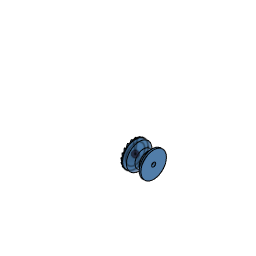
winch (Autodesk Fusion 360 design; units mm, degrees)
Autodesk Fusion 360 part; units mm, degrees
ref_plane "WorkPlane1" through (57.6974, -22.6085, 21.97) normal (-1, 0, 0) x (0, -1, 0)
sketch "Sketch1" plane through (57.6974, -45.4789, 40.4785) normal (-1, 0, 0) x (0, 1, 0)
  circle A0 centre (0, 0) radius 15
  line L0 (0, 0) -> (-2.3758, -15)
  line L1 (-2.3758, -15) -> (2.3758, -15)
  line L2 (2.3758, -15) -> (0, 0)
  circle A1 centre (0, 0) radius 11.1
  dimension "d113" = 30
  dimension "d114" = 18
  constraint coincident A0.centre L0.start
  constraint horizontal L1
  constraint tangent A0 L1
  constraint equal L0 L2
  measures "d113" diameter of A0
  measures "d114" angle of L0 L2
sketch "Sketch3" plane through (57.6974, -45.4789, 40.4785) normal (-1, 0, 0) x (0, 1, 0)
extrude "Extrude1" add sketch "Sketch1" against normal blind 7 contours A0 L0 L2 A1 | A0 L0 L2 A1 makes body 1
ref_plane "WorkPlane2" through (61.033, -45.4789, 55.4785) normal (0, 0, 1) x (0, 1, 0)
extrude "Extrude2" add sketch "Sketch1" along normal blind 2.1974 separate body contours A0 L0 L2 A1 picked at (1.2951, -12.322) makes body 2
sketch "Sketch2" plane through (36.883, -45.4789, 55.4785) normal (0, 0, 1) x (1, 0, 0)
  line L0 (20.8144, 2.3465) -> (18.617, 2.3465) construction
  line L1 (18.617, 2.3465) -> (18.617, -2.3465) construction
  line L2 (18.617, -2.3465) -> (20.8144, -2.3465) construction
  line L3 (18.617, 2.3465) -> (20.8144, -2.3465)
  line L4 (20.8144, -2.3465) -> (18.617, -2.3465)
  line L5 (18.617, -2.3465) -> (18.617, 2.3465)
  line L6 (20.8144, 2.3465) -> (20.8144, -2.3465)
  constraint coincident L0.end L1.start
  constraint coincident L2.end L3.end
  constraint coincident L1.end L2.start
extrude "Extrude3" cut sketch "Sketch2" against normal blind 10 bodies 2
pattern_circular "C-Pattern1" count 20 over 360 about axis through (57.6974, -45.4789, 40.4785) along (1, 0, 0) of bodies 2 makes body 3 at (56.5987, -49.3076, 52.2619) makes body 4 at (56.5987, -52.7615, 50.5021) makes body 5 at (56.5987, -55.5025, 47.761) makes body 6 at (56.5987, -57.2624, 44.3071) makes body 7 at (56.5987, -57.8688, 40.4785) makes body 8 at (56.5987, -57.2624, 36.6498) makes body 9 at (56.5987, -55.5025, 33.1959) makes body 10 at (56.5987, -52.7615, 30.4548) makes body 11 at (56.5987, -49.3076, 28.695) makes body 12 at (56.5987, -45.4789, 28.0886) makes body 13 at (56.5987, -41.6502, 28.695) makes body 14 at (56.5987, -38.1963, 30.4548) makes body 15 at (56.5987, -35.4553, 33.1959) makes body 16 at (56.5987, -33.6954, 36.6498) makes body 17 at (56.5987, -33.089, 40.4785) makes body 18 at (56.5987, -33.6954, 44.3071) makes body 19 at (56.5987, -35.4553, 47.761) makes body 20 at (56.5987, -38.1963, 50.5021) makes body 21 at (56.5987, -41.6502, 52.2619)
combine "Combine1" operation add target body 1 tool bodies 11 7 8 6 5 9 10 2 12 3 4 19 14 17 21 13 15 16 20 18
sketch "Sketch3 (1)" plane through (64.6974, 0, 0) normal (1, 0, 0) x (0, 1, 0)
  circle A0 centre (-45.4789, 40.4785) radius 11.1
  circle A1 centre (-45.4789, 40.4785) radius 15
  circle A2 centre (-45.4789, 40.4785) radius 4.1
  dimension "d144" = 8.2
  constraint concentric A0 A2
  measures "d144" diameter of A2
extrude "Extrude4" add sketch "Sketch3 (1)" along normal blind 2.1974 contours A0 | A1 bodies 1
sketch "Sketch4" plane through (66.8948, 0, 0) normal (1, 0, 0) x (0, 1, 0)
  circle A0 centre (-45.4789, 40.4785) radius 4.1
  circle A1 centre (-45.4789, 40.4785) radius 15
  circle A2 centre (-45.4789, 40.4785) radius 15
  constraint concentric A0 A2
extrude "Extrude5" add sketch "Sketch4" along normal blind 12.4077 contours A0 | A1 A2 bodies 1
sketch "Sketch6" plane through (-60, 55, 55.5) normal (0, 0, 1) x (-1, 0, 0)
  line L0 (-47.5194, 41.9) -> (-47.5194, 39.034)
  arc A0 (-47.5194, 39.034) -> (-47.5354, 41.9) centre (-45.4789, 40.4785) ccw
  line L1 (-47.5354, 41.9) -> (-47.5194, 41.9)
  circle A1 centre (-45.4789, 40.4785) radius 2.7
  dimension "d157" = 5.4
  constraint concentric A0 A1
  measures "d157" diameter of A1
extrude "Extrude6" cut sketch "Sketch6" against normal blind 1.6052 contours L0 A0 L1 | A1 bodies 1
ref_plane "WorkPlane3" through (76.7969, -60.4789, 40.4785) normal (0, -1, 0) x (0, 0, 1)
ref_plane "WorkPlane4" through (76.7969, -45.4789, 40.4785) normal (0, -1, 0) x (0, 0, 1)
sketch "Sketch5" plane through (52.6469, -45.4789, 40.4785) normal (0, -1, 0) x (1, 0, 0)
  line L0 (26.6556, -15) -> (26.6556, 15) construction
  line L1 (5.0505, -13.3651) -> (2.8531, -13.3651) construction
  ellipse E0 centre (3.9518, 0) end of major axis (6.634, -14.9547) minor radius 6.5947 (2.8531, -13.3651) -> (5.0505, -14.8153) ccw
  line L2 (5.0505, -14.8153) -> (2.8531, -14.8153) construction
  ellipse E1 centre (3.9518, 0) end of major axis (3.9518, -15) minor radius 7.0235 (2.8531, -14.8153) -> (5.0505, -14.8153) ccw
  line L3 (5.0505, -14.8153) -> (2.8531, -14.8153) construction
  ellipse E2 centre (3.9518, 0) end of major axis (1.2695, -14.9547) minor radius 6.5947 (2.8531, -14.8153) -> (5.0505, -13.3651) ccw
  line L4 (5.0505, -13.3651) -> (2.8531, -13.3651) construction
  ellipse E3 centre (3.9518, 0) end of major axis (-0.7754, -14.9093) minor radius 5.4493 (2.8531, -13.3651) -> (5.0505, -10.6066) ccw
  line L5 (5.0505, -10.6066) -> (2.8531, -10.6066) construction
  ellipse E4 centre (3.9518, 0) end of major axis (-2.1014, -14.9303) minor radius 3.8437 (2.8531, -10.6066) -> (5.0505, -6.8099) ccw
  line L6 (5.0505, -6.8099) -> (2.8531, -6.8099) construction
  ellipse E5 centre (3.9518, 0) end of major axis (-2.8363, -14.9777) minor radius 1.9798 (2.8531, -6.8099) -> (5.0505, -2.3465) ccw
  line L7 (5.0505, -2.3465) -> (2.8531, -2.3465) construction
  line L8 (2.8531, -2.3465) -> (5.0505, 2.3465) construction
  line L9 (5.0505, 2.3465) -> (2.8531, 2.3465) construction
  ellipse E6 centre (3.9518, 0) end of major axis (-2.8363, -14.9777) minor radius 1.9798 (5.0505, 6.8099) -> (2.8531, 2.3465) ccw
  line L10 (5.0505, 6.8099) -> (2.8531, 6.8099) construction
  ellipse E7 centre (3.9518, 0) end of major axis (10.0049, 14.9303) minor radius 3.8437 (5.0505, 10.6066) -> (2.8531, 6.8099) ccw
  line L11 (5.0505, 10.6066) -> (2.8531, 10.6066) construction
  ellipse E8 centre (3.9518, 0) end of major axis (8.679, 14.9093) minor radius 5.4493 (5.0505, 13.3651) -> (2.8531, 10.6066) ccw
  line L12 (5.0505, 13.3651) -> (2.8531, 13.3651) construction
  ellipse E9 centre (3.9518, 0) end of major axis (6.634, 14.9547) minor radius 6.5947 (5.0505, 14.8153) -> (2.8531, 13.3651) ccw
  line L13 (5.0505, 14.8153) -> (2.8531, 14.8153) construction
  ellipse E10 centre (3.9518, 0) end of major axis (3.9518, 15) minor radius 7.0235 (5.0505, 14.8153) -> (2.8531, 14.8153) ccw
  line L14 (5.0505, 14.8153) -> (2.8531, 14.8153) construction
  ellipse E11 centre (3.9518, 0) end of major axis (1.2695, 14.9547) minor radius 6.5947 (5.0505, 13.3651) -> (2.8531, 14.8153) ccw
  line L15 (5.0505, 13.3651) -> (2.8531, 13.3651) construction
  ellipse E12 centre (3.9518, 0) end of major axis (-0.7754, 14.9093) minor radius 5.4493 (5.0505, 10.6066) -> (2.8531, 13.3651) ccw
  line L16 (5.0505, 10.6066) -> (2.8531, 10.6066) construction
  ellipse E13 centre (3.9518, 0) end of major axis (-2.1014, 14.9303) minor radius 3.8437 (5.0505, 6.8099) -> (2.8531, 10.6066) ccw
  line L17 (5.0505, 6.8099) -> (2.8531, 6.8099) construction
  ellipse E14 centre (3.9518, 0) end of major axis (-2.8363, 14.9777) minor radius 1.9798 (5.0505, 2.3465) -> (2.8531, 6.8099) ccw
  line L18 (5.0505, 2.3465) -> (2.8531, 2.3465) construction
  line L19 (5.0505, -2.3465) -> (2.8531, 2.3465) construction
  line L20 (5.0505, -2.3465) -> (2.8531, -2.3465) construction
  ellipse E15 centre (3.9518, 0) end of major axis (-2.8363, 14.9777) minor radius 1.9798 (2.8531, -2.3465) -> (5.0505, -6.8099) ccw
  line L21 (5.0505, -6.8099) -> (2.8531, -6.8099) construction
  ellipse E16 centre (3.9518, 0) end of major axis (10.0049, -14.9303) minor radius 3.8437 (2.8531, -6.8099) -> (5.0505, -10.6066) ccw
  line L22 (5.0505, -10.6066) -> (2.8531, -10.6066) construction
  ellipse E17 centre (3.9518, 0) end of major axis (8.679, -14.9093) minor radius 5.4493 (2.8531, -10.6066) -> (5.0505, -13.3651) ccw
  line L23 (9.6556, 15) -> (24.6556, 15)
  line L24 (24.6556, 15) -> (24.6556, 10)
  line L25 (24.6556, 10) -> (9.6556, 10)
  line L26 (9.6556, 10) -> (9.6556, 15)
  line L27 (9.6556, 15) -> (14.6556, 10)
  line L28 (14.6556, 10) -> (19.6556, 10)
  line L29 (19.6556, 10) -> (24.6556, 15)
  dimension "d152" = 2
  dimension "d153" = 15
  dimension "d154" = 5
  dimension "d155" = 5
  constraint horizontal L23
  constraint vertical L24
  constraint horizontal L25
  constraint vertical L26
  constraint coincident L0.end L23
  constraint coincident L25 L27.end
  constraint coincident L25 L28.end
  constraint equal L27 L29
  measures "d152" distance of L0.end L24
  measures "d153" distance of L23.start L23.end
  measures "d154" distance of L23.end L24.end
  measures "d155" distance of L27.end L28.end
revolve "Revolve1" cut sketch "Sketch5" angle 360 about axis through (66.8948, -45.4789, 40.4785) along (-1, 0, 0) contours L23 L25 L27 L28 L29 bodies 1
sketch "Sketch7" plane through (79.3026, 0, 0) normal (1, 0, 0) x (0, 1, 0)
  circle A0 centre (-45.4789, 40.4785) radius 15
  circle A1 centre (-45.4789, 40.4785) radius 2.35
  dimension "d161" = 4.7
  constraint concentric A0 A1
  measures "d161" diameter of A1
extrude "Extrude7" cut sketch "Sketch7" against normal blind 3 contours A1 bodies 1
equation "d112 = -gearThickness"
equation "d113 = gearDiameter"
equation "d114 = gearToothCenterAngle"
equation "d115 = -gearToothDepth"
equation "d123 = -gearWinchBaseThickness"
equation "d126 = gearToothThickness"
equation "d130 = gearToothNumber"
equation "d144 = bearingHoleDiameter + tolerance"
equation "d145 = gearToothThickness"
equation "d148 = pullyWidth - ( 3 * gearToothThickness )"
equation "d151 = gearDiameter / -2"
equation "d152 = pulleyWallThickness"
equation "d153 = creviceWidth + winchGap"
equation "d154 = creviceDepth"
equation "d157 = stepperMotorShaftDiameter + ( tolerance * 2 )"
equation "d161 = screwDiameter + tolerance * 2"
equation "d162 = -springDepth"
equation "tolerance = 0.2 mm"
equation "gearDiameter = 30 mm"
equation "gearToothThickness = gearToothWidth * tan(gearToothAngle)"
equation "gearToothNumber = 20"
equation "gearToothWidth = ( gearDiameter / 2 ) * gearToothCenterAngleRad / 1 rad"
equation "gearBaseThickness = 9 mm"
equation "gearToothAngle = 25 deg"
equation "gearToothCenterAngle = ( 360 / gearToothNumber ) * 1 deg"
equation "gearToothCenterAngleRad = gearToothCenterAngle"
equation "gearToothDepth = 4 mm - ( tolerance / 2 )"
equation "pullyWidth = ( pulleyWallThickness * 2 ) + creviceWidth + winchGap"
equation "creviceDepth = 5 mm"
equation "creviceWidth = 10 mm"
equation "pulleyWallThickness = 2 mm"
equation "springDepth = 3 mm"
equation "stepperMotorShaftDiameter = 5 mm"
equation "gearThickness = gearToothThickness + gearBaseThickness"
equation "gearWinchBaseThickness = bearingWidth"
equation "bearingWidth = 7 mm"
equation "bearingHoleDiameter = 8 mm"
equation "winchGap = 5 mm"
equation "screwDiameter = 4.3 mm"
